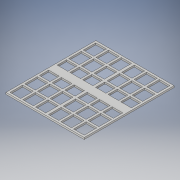
# Autodesk Inventor part: 4 Tape Measures Holder V2
Saved by Autodesk Inventor 2019 (Build 230136000, 136)
## iProperties
Created: 2018-12-28
Part Number: 4 Tape Measures Holder V2
Material: Generic
Document SubType Name: Modeling
Designer: ashle
Density: 1 g/cm^3
Appearance: Default
Author: ashle
Autodesk Inventor part; units mm, degrees
ref_plane "YZ Plane" through (0, 0, 0) normal (1, 0, 0) x (0, 1, 0)
ref_plane "XZ Plane" through (0, 0, 0) normal (0, 1, 0) x (-1, 0, 0)
ref_plane "XY Plane" through (0, 0, 0) normal (0, 0, 1) x (1, 0, 0)
sketch "Sketch1" plane through (0, 0, 0) normal (0, 1, 0) x (-1, 0, 0)
  line L0 (108, 131) -> (-108, 131)
  line L1 (-108, 131) -> (-108, 125)
  line L2 (-108, 125) -> (108, 125)
  line L3 (108, 125) -> (108, 131)
  line L4 (0, 5131.2687) -> (0, -192.5797)
  line L5 (108, 4620.3571) -> (108, -4424.6448)
  line L6 (-108, 163.2413) -> (-108, -192.5797)
  line L7 (-159.6212, -125) -> (141.3387, -125)
  line L8 (141.3387, 125) -> (-159.6212, 125)
  line L9 (-108, 88.3333) -> (-108, 82.3333)
  line L10 (108, 88.3333) -> (-108, 88.3333)
  line L11 (-108, 82.3333) -> (108, 82.3333)
  line L12 (108, 82.3333) -> (108, 88.3333)
  line L13 (-108, 45.6667) -> (-108, 39.6667)
  line L14 (108, 45.6667) -> (-108, 45.6667)
  line L15 (-108, 39.6667) -> (108, 39.6667)
  line L16 (108, 39.6667) -> (108, 45.6667)
  line L17 (-108, -12.5) -> (108, -12.5)
  line L18 (108, -12.5) -> (108, 12.5)
  line L19 (108, 12.5) -> (-108, 12.5)
  line L20 (-108, 12.5) -> (-108, -12.5)
  line L21 (-108, -12.5) -> (108, 12.5) construction
  line L22 (108, -12.5) -> (-108, 12.5) construction
  line L23 (-4, -131) -> (4, -131)
  line L24 (4, -131) -> (4, 131)
  line L25 (4, 131) -> (-4, 131)
  line L26 (-4, 131) -> (-4, -131)
  line L27 (-4, -131) -> (4, 131) construction
  line L28 (4, -131) -> (-4, 131) construction
  line L29 (3750.9383, 0) -> (-5642.9813, 0)
  line L30 (108, -131) -> (-108, -131)
  line L31 (-108, -131) -> (-108, -125)
  line L32 (-108, -125) -> (108, -125)
  line L33 (108, -125) -> (108, -131)
  line L34 (-108, -88.3333) -> (-108, -82.3333)
  line L35 (108, -88.3333) -> (-108, -88.3333)
  line L36 (-108, -82.3333) -> (108, -82.3333)
  line L37 (108, -82.3333) -> (108, -88.3333)
  line L38 (-108, -45.6667) -> (-108, -39.6667)
  line L39 (108, -45.6667) -> (-108, -45.6667)
  line L40 (-108, -39.6667) -> (108, -39.6667)
  line L41 (108, -39.6667) -> (108, -45.6667)
  line L42 (114, 131) -> (108, 131)
  line L43 (108, 131) -> (108, -131)
  line L44 (108, -131) -> (114, -131)
  line L45 (114, -131) -> (114, 131)
  line L46 (71, 131) -> (71, -131)
  line L47 (77, -131) -> (77, 131)
  line L48 (77, 131) -> (71, 131)
  line L49 (71, -131) -> (77, -131)
  line L50 (34, 131) -> (34, -131)
  line L51 (40, -131) -> (40, 131)
  line L52 (40, 131) -> (34, 131)
  line L53 (34, -131) -> (40, -131)
  line L54 (-114, 131) -> (-108, 131)
  line L55 (-108, 131) -> (-108, -131)
  line L56 (-108, -131) -> (-114, -131)
  line L57 (-114, -131) -> (-114, 131)
  line L58 (-71, 131) -> (-71, -131)
  line L59 (-77, -131) -> (-77, 131)
  line L60 (-77, 131) -> (-71, 131)
  line L61 (-71, -131) -> (-77, -131)
  line L62 (-34, 131) -> (-34, -131)
  line L63 (-40, -131) -> (-40, 131)
  line L64 (-40, 131) -> (-34, 131)
  line L65 (-34, -131) -> (-40, -131)
  line L66 (-159.6212, -192.5797) -> (141.3387, -192.5797)
  line L67 (141.3387, -192.5797) -> (141.3387, 163.2413)
  line L68 (141.3387, 163.2413) -> (-159.6212, 163.2413)
  line L69 (-159.6212, 163.2413) -> (-159.6212, -192.5797)
  point P0 (0, 0)
  point P1 (-71, 131)
  dimension "d0" = 216
  dimension "d1" = 6
  dimension "d5" = 108
  dimension "d6" = 125
  dimension "d7" = 250
  dimension "d10" = 42.6667
  dimension "d15" = 25
  dimension "d16" = 8
  dimension "d19" = 79.3333
  dimension "d20" = 79.3333
  dimension "d21" = 6
  dimension "d24" = 37
  dimension "d29" = 68
  dimension "d30" = 68
  dimension "d32" = 37
  dimension "d33" = 42.6667
  dimension "d36" = 6
  dimension "d37" = 6
  constraints: 140 end point, 28 symmetric about line, 10 parallel, 9 horizontal, 8 collinear, 7 point on line, 5 perpendicular, 4 midpoint, 4 vertical, 36 other
  measures "d0" distance of L0.start L0.end
  measures "d1" distance of L2.end L0.start
  measures "d5" distance from line of point (0, 0) L1
  measures "d6" distance from line of point (0, 0) L2
  measures "d7" distance between parallel lines of L7 L8
  measures "d10" distance of L0.end L9.start
  measures "d15" distance between parallel lines of L17 L19
  measures "d16" distance between parallel lines of L26 L24
  measures "d19" distance between parallel lines of L14 L2
  measures "d20" distance between parallel lines of L40 L15
  measures "d21" distance of L42.start L42.end
  measures "d24" distance of L42.end L46.start
  measures "d29" distance between parallel lines of L43 L51
  measures "d30" distance between parallel lines of L62 L50
  measures "d32" distance between parallel lines of L58 L62
  measures "d33" distance between parallel lines of L40 L36
  measures "d36" distance between parallel lines of L35 L36
  measures "d37" distance between parallel lines of L59 L58
extrude "Extrusion1" add sketch "Sketch1" along normal blind 5 contours L3 L2 L47 L0 | L42 L45 L8 L3 | L47 L2 L46 L0 | L8 L45 L29 L5 | L46 L2 L51 L0 | L47 L10 L46 L2 | L5 L11 L47 L10 | L51 L2 L50 L0 | L47 L11 L46 L10 | L45 L7 L5 L29 | L4 L2 L26 L0 | L0 L24 L2 L4 | L50 L2 L24 L0 | L51 L10 L50 L2 | L46 L11 L51 L10 | L47 L14 L46 L11 | L5 L15 L47 L14 | L29 L47 L19 L5 | L5 L17 L47 L29 | L45 L44 L5 L7 | L26 L2 L62 L0 | L4 L10 L26 L2 | L2 L24 L10 L4 | L0 L59 L2 L1 | L1 L8 L57 L54 | L51 L11 L50 L10 | L47 L15 L46 L14 | L47 L17 L46 L29 | L29 L46 L19 L47 | L5 L30 L47 L7 | L62 L2 L63 L0 | L10 L24 L11 L4 | L4 L11 L26 L10 | L0 L58 L2 L59 | L6 L29 L57 L8 | L50 L11 L24 L10 | L51 L14 L50 L11 | L46 L15 L51 L14 | L47 L19 L46 L15 | L5 L39 L47 L40 | L47 L40 L46 L17 | L46 L17 L51 L29 | L29 L51 L19 L46 | L35 L47 L36 L5 | L47 L30 L46 L7 | L7 L46 L35 L47 | L63 L2 L58 L0 | L62 L10 L63 L2 | L26 L11 L62 L10 | L11 L24 L14 L4 | L4 L14 L26 L11 | L2 L58 L10 L59 | L10 L59 L11 L6 | L51 L15 L50 L14 | L47 L39 L46 L40 | L51 L17 L50 L29 | L29 L50 L19 L51 | L35 L46 L36 L47 | L46 L30 L51 L7 | L62 L11 L63 L10 | L14 L24 L15 L4 | L4 L15 L26 L14 | L10 L58 L11 L59 | L29 L6 L7 L57 | L50 L15 L24 L14 | L51 L19 L50 L15 | L47 L36 L46 L39 | L46 L39 L51 L40 | L51 L40 L50 L17 | L50 L17 L24 L29 | L29 L24 L19 L50 | L35 L51 L36 L46 | L51 L30 L50 L7 | L7 L50 L35 L51 | L63 L11 L58 L10 | L62 L14 L63 L11 | L26 L15 L62 L14 | L15 L24 L19 L4 | L4 L19 L26 L15 | L11 L58 L14 L59 | L14 L59 L15 L6 | L29 L59 L17 L6 | L6 L19 L59 L29 | L7 L6 L56 L57 | L23 L26 L7 L4 | L4 L7 L24 L23 | L51 L39 L50 L40 | L29 L4 L19 L24 | L24 L17 L4 L29 | L35 L50 L36 L51 | L50 L30 L24 L7 | L62 L15 L63 L14 | L4 L29 L26 L19 | L14 L58 L15 L59 | L59 L19 L58 L29 | L29 L58 L17 L59 | L7 L59 L30 L6 | L7 L26 L35 L4 | L4 L35 L24 L7 | L30 L62 L7 L26 | L51 L36 L50 L39 | L50 L39 L24 L40 | L24 L40 L4 L17 | L4 L17 L26 L29 | L35 L24 L36 L50 | L63 L15 L58 L14 | L62 L19 L63 L15 | L26 L29 L62 L19 | L15 L58 L19 L59 | L40 L59 L39 L6 | L17 L58 L40 L59 | L58 L19 L63 L29 | L29 L63 L17 L58 | L6 L36 L59 L35 | L59 L35 L58 L7 | L7 L58 L30 L59 | L35 L26 L36 L4 | L4 L36 L24 L35 | L30 L63 L7 L62 | L24 L39 L4 L40 | L4 L40 L26 L17 | L26 L17 L62 L29 | L62 L29 L63 L19 | L40 L58 L39 L59 | L29 L62 L17 L63 | L59 L36 L58 L35 | L7 L63 L30 L58 | L36 L26 L39 L4 | L4 L39 L24 L36 | L35 L62 L36 L26 | L7 L63 L35 L62 | L4 L39 L26 L40 | L39 L58 L36 L59 | L40 L63 L39 L58 | L17 L62 L40 L63 | L58 L36 L63 L35 | L35 L63 L36 L62 | L26 L39 L62 L40 | L40 L62 L39 L63 | L36 L63 L39 L62
equation "\"d0\" = 2 * d5"
equation "\"d7\" = 2 * d6"
equation "\"d10\" = 0.166667 * d7 + 0.166667 * d1"
equation "\"d20\" = d19"
equation "\"d21\" = d1"
equation "\"d24\" = 0.166667 * d0 + 0.166667 * d21"
equation "\"d30\" = d29"
body "Solid1"
